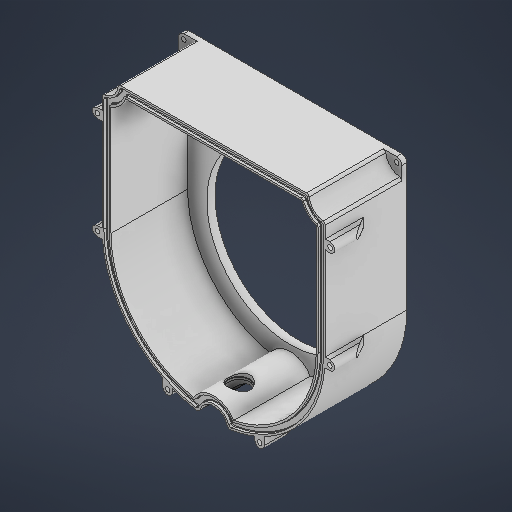
# Autodesk Inventor part: reservoir_cap
Saved by Autodesk Inventor 2026.2 (Build 302298000, 298)
## iProperties
Created: 2026-04-07
Part Number: reservoir_cap
Material: Generic
Document SubType Name: Modeling
Designer: Tathagata Sikdar
Density: 1 g/cm^3
Appearance: Default
Author: Tathagata Sikdar
Autodesk Inventor part; units mm, degrees
note: some values were not read from the file. Chosen so that the rebuilt part matches the saved one: direction of "Hole2".
ref_plane "Work Plane1" through (0, 0, 0) normal (0, 0, 1) x (1, 0, 0)
sketch "Sketch1" plane through (0, 0, 0) normal (0, 0, 1) x (1, 0, 0)
  arc A0 (-87.3944, 0) -> (87.3944, 0) centre (0, 0) ccw projected
  line L0 (-87.3944, 0) -> (-87.3944, 100.0128) projected
  arc A1 (-83.3944, 104.0128) -> (-87.3944, 100.0128) centre (-83.3944, 100.0128) ccw projected
  line L1 (-83.3944, 104.0128) -> (83.3944, 104.0128) projected
  arc A2 (87.3944, 100.0128) -> (83.3944, 104.0128) centre (83.3944, 100.0128) ccw projected
  line L2 (87.3944, 100.0128) -> (87.3944, 0) projected
  circle A3 centre (83.3944, 100.0128) radius 1.85 projected
  circle A4 centre (-83.3944, 100.0128) radius 1.85 projected
  circle A5 centre (0, -83.8944) radius 1.85 projected
  circle A6 centre (0, 0) radius 68.3944 construction
  arc A7 (10, -69.6805) -> (-10, -69.6805) centre (0, 0) ccw construction
  arc A8 (-39.9607, -69.7596) -> (-10, -69.6805) centre (-25.049, -43.7281) ccw construction
  arc A9 (-80.3944, 0) -> (-39.9607, -69.7596) centre (0, 0) ccw construction
  line L3 (-80.3944, 87.0128) -> (-80.3944, 0) construction
  line L4 (-70.3944, 97.0128) -> (-80.3944, 87.0128) construction
  line L5 (70.3944, 97.0128) -> (-70.3944, 97.0128) construction
  line L6 (80.3944, 87.0128) -> (70.3944, 97.0128) construction
  line L7 (80.3944, 0) -> (80.3944, 87.0128) construction
  arc A10 (39.9607, -69.7596) -> (80.3944, 0) centre (0, 0) ccw construction
  arc A11 (10, -69.6805) -> (39.9607, -69.7596) centre (25.049, -43.7281) ccw construction
  arc A12 (14.16, -70.0577) -> (-14.16, -70.0577) centre (0, 0) ccw
  arc A13 (42.1402, -68.1714) -> (80.1444, 0) centre (0, 0) ccw
  line L8 (80.1444, 0) -> (80.1444, 86.9092)
  line L9 (80.1444, 86.9092) -> (70.2909, 96.7628)
  line L10 (70.2909, 96.7628) -> (-70.2909, 96.7628)
  line L11 (-70.2909, 96.7628) -> (-80.1444, 86.9092)
  line L12 (-80.1444, 86.9092) -> (-80.1444, 0)
  arc A14 (-80.1444, 0) -> (-42.1402, -68.1714) centre (0, 0) ccw
  circle A15 centre (0, 0) radius 67.3144
  arc A16 (14.16, -70.0577) -> (42.1402, -68.1714) centre (26.3661, -42.6532) ccw
  arc A17 (-42.1402, -68.1714) -> (-14.16, -70.0577) centre (-26.3661, -42.6532) ccw
  circle A18 centre (0, 0) radius 65.3144
  arc A19 (17.5846, -71.3391) -> (-17.5846, -71.3391) centre (0, 0) ccw
  line L13 (-78.1444, 0) -> (-78.1444, 86.0808)
  line L14 (-78.1444, 86.0808) -> (-69.4624, 94.7628)
  line L15 (-69.4624, 94.7628) -> (69.4624, 94.7628)
  line L16 (69.4624, 94.7628) -> (78.1444, 86.0808)
  line L17 (78.1444, 86.0808) -> (78.1444, 0)
  arc A20 (41.0886, -66.4701) -> (78.1444, 0) centre (0, 0) ccw
  arc A21 (21.565, -70.2385) -> (41.0886, -66.4701) centre (26.3661, -42.6532) ccw
  arc A22 (21.565, -70.2385) -> (-21.565, -70.2385) centre (0, 0) ccw
  arc A23 (-41.0886, -66.4701) -> (-21.565, -70.2385) centre (-26.3661, -42.6532) ccw
  arc A24 (-78.1444, 0) -> (-41.0886, -66.4701) centre (0, 0) ccw
  point P0 (-21.565, -70.2385)
  point P1 (21.565, -70.2385)
  dimension "GasketWidth" = 4.16
  dimension "d1" = 2
  dimension "d2" = -1.08
  dimension "Tolerance" = 0.25
  dimension "d4" = 2
  dimension "d5" = 4.16
  dimension "d6" = 4.16
  dimension "d7" = 2
  dimension "d10" = 2
  constraints: 24 point on circle, 20 end point, 13 centre point, 2 equal radius, 2 tangent, 1 coincident, 15 other
  measures "GasketWidth" radial gap between concentric circles of A12 A15
  measures "d1" radial gap between concentric circles of A7 A6
  measures "d2" radial gap between concentric circles of A6 A15
  measures "Tolerance" distance between parallel lines of L5 L10
  measures "d4" radial gap between concentric circles of A15 A18
  measures "d5" horizontal distance of A7.start A12.start
  measures "d6" horizontal distance of A7.end A12.end
  measures "d7" radial gap between concentric circles of A19 A12
  measures "d10" distance between parallel lines of L12 L13
extrude "Extrusion1" add sketch "Sketch1" against normal blind 2.38 contours A12 A17 A19 A16 | A19 A21 A20 L17 L16 L15 L14 L13 A24 A23 A17 A14 L12 L11 L10 L9 L8 A13 A16 | A15
ref_plane "Work Plane2" through (0, 0, 0) normal (0, 0, 1) x (1, 0, 0)
sketch "Sketch2" plane through (0, 0, 0) normal (0, 0, 1) x (1, 0, 0)
  arc A0 (-87.3944, 0) -> (87.3944, 0) centre (0, 0) ccw projected
  line L0 (-87.3944, 0) -> (-87.3944, 100.0128) projected
  arc A1 (-83.3944, 104.0128) -> (-87.3944, 100.0128) centre (-83.3944, 100.0128) ccw projected
  line L1 (-83.3944, 104.0128) -> (83.3944, 104.0128) projected
  arc A2 (87.3944, 100.0128) -> (83.3944, 104.0128) centre (83.3944, 100.0128) ccw projected
  line L2 (87.3944, 100.0128) -> (87.3944, 0) projected
  circle A3 centre (83.3944, 100.0128) radius 1.85 projected
  circle A4 centre (-83.3944, 100.0128) radius 1.85 projected
  circle A5 centre (0, -83.8944) radius 1.85 projected
  circle A6 centre (0, 0) radius 65.3144 projected
extrude "Extrusion2" add sketch "Sketch2" along normal blind 4
fillet "Fillet1" radius 0.4 2 edges at (-67.3144, 0, 0) (0, 71.4744, 0)
sketch "Sketch3" plane through (0, 0, 4) normal (0, 0, 1) x (1, 0, 0)
  arc A0 (-87.3944, 0) -> (87.3944, 0) centre (0, 0) ccw construction
  line L0 (-87.3944, 100.0128) -> (-87.3944, 0) construction
  arc A1 (-83.3944, 104.0128) -> (-87.3944, 100.0128) centre (-83.3944, 100.0128) ccw construction
  line L1 (83.3944, 104.0128) -> (-83.3944, 104.0128) construction
  arc A2 (87.3944, 100.0128) -> (83.3944, 104.0128) centre (83.3944, 100.0128) ccw construction
  line L2 (87.3944, 0) -> (87.3944, 100.0128) construction
  line L3 (-87.3944, 0) -> (-87.3944, 91.2848)
  line L4 (-74.6665, 104.0128) -> (74.6665, 104.0128)
  line L5 (87.3944, 91.2848) -> (87.3944, 0)
  arc A3 (11.1256, -86.6834) -> (87.3944, 0) centre (0, 0) ccw
  arc A4 (-87.3944, 0) -> (-11.1256, -86.6834) centre (0, 0) ccw
  circle A5 centre (0, -83.8944) radius 1.85 construction
  arc A6 (74.6665, 104.0128) -> (87.3944, 91.2848) centre (87.3944, 104.0128) ccw
  arc A7 (-87.3944, 91.2848) -> (-74.6665, 104.0128) centre (-87.3944, 104.0128) ccw
  arc A8 (11.1256, -86.6834) -> (-11.1256, -86.6834) centre (0, -88.1113) ccw
  line L6 (-74.6665, 104.0128) -> (74.6665, 104.0128)
  arc A9 (74.6665, 104.0128) -> (87.3944, 91.2848) centre (87.3944, 104.0128) ccw
  line L7 (87.3944, 91.2848) -> (87.3944, 0)
  arc A10 (11.1256, -86.6834) -> (87.3944, 0) centre (0, 0) ccw
  arc A11 (11.1256, -86.6834) -> (-11.1256, -86.6834) centre (0, -88.1113) ccw
  arc A12 (-87.3944, 0) -> (-11.1256, -86.6834) centre (0, 0) ccw
  line L8 (-87.3944, 0) -> (-87.3944, 91.2848)
  arc A13 (-87.3944, 91.2848) -> (-74.6665, 104.0128) centre (-87.3944, 104.0128) ccw
  arc A14 (15.6866, -78.8492) -> (-15.6866, -78.8492) centre (0, -88.1113) ccw
  arc A15 (-80.3944, 0) -> (-15.6866, -78.8492) centre (0, 0) ccw
  arc A16 (15.6866, -78.8492) -> (80.3944, 0) centre (0, 0) ccw
  line L9 (80.3944, 0) -> (80.3944, 85.5685)
  arc A17 (68.9502, 97.0128) -> (80.3944, 85.5685) centre (87.3944, 104.0128) ccw
  line L10 (68.9502, 97.0128) -> (-68.9502, 97.0128)
  arc A18 (-80.3944, 85.5685) -> (-68.9502, 97.0128) centre (-87.3944, 104.0128) ccw
  line L11 (-80.3944, 85.5685) -> (-80.3944, 0)
  point P0 (0, -76.8944)
  point P1 (-78.3944, 95.0128)
  point P2 (78.3944, 95.0128)
  dimension "d14" = 7
  dimension "d15" = 5
  dimension "d16" = 5
  dimension "d17" = 7
  dimension "d18" = 7
  dimension "d19" = 7
  dimension "d20" = 7
  dimension "d21" = 7
  dimension "d22" = 7
  constraints: 34 point on circle, 18 end point, 15 centre point, 7 concentric, 4 line through centre, 2 tangent, 2 vertical, 1 collinear, 1 horizontal, 1 vertical alignment, 13 other
  measures "d14" distance of A5.centre point (0, -76.894)
  measures "d15" horizontal distance of A1.centre point (-78.394, 95.013)
  measures "d16" horizontal distance of A2.centre point (78.394, 95.013)
  measures "d17" radial gap between concentric circles of A6 A17
  measures "d18" radial gap between concentric circles of A13 A18
  measures "d19" distance between parallel lines of L6 L10
  measures "d20" distance between parallel lines of L8 L11
  measures "d21" distance between parallel lines of L2 L9
  measures "d22" radial gap between concentric circles of A8 A14
extrude "Extrusion3" add sketch "Sketch3" along normal blind 60
sketch "Sketch4" plane through (0, 0, 64) normal (0, 0, 1) x (1, 0, 0)
  circle A0 centre (-91.1444, -3.7152) radius 1.85
  arc A1 (-91.1444, 0.0348) -> (-91.1444, -7.4652) centre (-91.1444, -3.7152) ccw
  circle A2 centre (91.0687, -3.7152) radius 1.85
  arc A3 (91.0687, -7.4652) -> (91.0687, 0.0348) centre (91.0687, -3.7152) ccw
  circle A4 centre (-36.0427, -83.7152) radius 1.85
  arc A5 (-39.7927, -83.7152) -> (-32.2927, -83.7152) centre (-36.0427, -83.7152) ccw
  circle A6 centre (36.0427, -83.7152) radius 1.85
  arc A7 (32.2927, -83.7152) -> (39.7927, -83.7152) centre (36.0427, -83.7152) ccw
  circle A8 centre (-91.1444, 76.2848) radius 1.85
  arc A9 (-91.1444, 80.0348) -> (-91.1444, 72.5348) centre (-91.1444, 76.2848) ccw
  circle A10 centre (91.1444, 76.2848) radius 1.85
  arc A11 (91.1444, 72.5348) -> (91.1444, 80.0348) centre (91.1444, 76.2848) ccw
  arc A12 (11.1256, -86.6834) -> (87.3944, 0) centre (0, 0) ccw projected
  line L0 (87.3944, 0) -> (87.3944, 91.2848) projected
  arc A13 (74.6665, 104.0128) -> (87.3944, 91.2848) centre (87.3944, 104.0128) ccw construction
  line L1 (74.6665, 104.0128) -> (-74.6665, 104.0128) construction
  arc A14 (-87.3944, 91.2848) -> (-74.6665, 104.0128) centre (-87.3944, 104.0128) ccw construction
  line L2 (-87.3944, 91.2848) -> (-87.3944, 0) projected
  arc A15 (-87.3944, 0) -> (-11.1256, -86.6834) centre (0, 0) ccw projected
  arc A16 (11.1256, -86.6834) -> (-11.1256, -86.6834) centre (0, -88.1113) ccw construction
  arc A17 (15.6866, -78.8492) -> (80.3944, 0) centre (0, 0) ccw construction
  arc A18 (15.6866, -78.8492) -> (-15.6866, -78.8492) centre (0, -88.1113) ccw construction
  arc A19 (-80.3944, 0) -> (-15.6866, -78.8492) centre (0, 0) ccw construction
  line L3 (-80.3944, 0) -> (-80.3944, 85.5685) construction
  arc A20 (-80.3944, 85.5685) -> (-68.9502, 97.0128) centre (-87.3944, 104.0128) ccw construction
  line L4 (-68.9502, 97.0128) -> (68.9502, 97.0128) construction
  arc A21 (68.9502, 97.0128) -> (80.3944, 85.5685) centre (87.3944, 104.0128) ccw construction
  line L5 (80.3944, 85.5685) -> (80.3944, 0) construction
  line L6 (87.3944, 0) -> (87.3944, 91.2848) construction
  line L7 (-87.3944, 91.2848) -> (-87.3944, 0) construction
  line L8 (-91.1444, 80.0348) -> (-87.3944, 80.0348)
  line L9 (-91.1444, 72.5348) -> (-87.3944, 72.5348)
  line L10 (-91.1444, 0.0348) -> (-87.3944, 0.0348)
  line L11 (-91.1444, -7.4652) -> (-87.075, -7.4652)
  line L12 (-39.7927, -83.7152) -> (-39.7927, -77.8095)
  line L13 (-32.2927, -83.7152) -> (-32.2927, -81.2094)
  line L14 (32.2927, -83.7152) -> (32.2927, -81.2094)
  line L15 (39.7927, -83.7152) -> (39.7927, -77.8095)
  line L16 (91.0687, 0.0348) -> (87.3944, 0.0348)
  line L17 (91.0687, -7.4652) -> (87.075, -7.4652)
  line L18 (91.1444, 80.0348) -> (87.3944, 80.0348)
  line L19 (91.1444, 72.5348) -> (87.3944, 72.5348)
  dimension "d25" = 3.7
  dimension "d27" = 3.7
  dimension "d29" = 3.7
  dimension "d31" = 3.7
  dimension "d33" = 3.7
  dimension "d34" = 7.5
  dimension "d35" = 3.7
  dimension "d37" = 15
  dimension "d38" = 80
  dimension "d39" = 80
  constraints: 24 end point, 18 point on circle, 16 tangent, 12 centre point, 10 point on line, 6 coincident, 6 parallel, 5 equal radius, 4 perpendicular, 3 horizontal alignment
  measures "d25" diameter of A0
  measures "d27" diameter of A2
  measures "d29" diameter of A4
  measures "d31" diameter of A6
  measures "d33" diameter of A8
  measures "d34" diameter of A9
  measures "d35" diameter of A10
  measures "d37" vertical distance of L2.start A8.centre
  measures "d38" distance of A8.centre A0.centre
  measures "d39" vertical distance of A0.centre A4.centre
extrude "Extrusion4" add sketch "Sketch4" against normal blind 30
sketch "Sketch5" plane through (0, 0, 34) normal (0, 0, -1) x (-1, 0, 0)
  line L0 (87.3944, 72.5348) -> (91.1444, 72.5348) projected
  arc A0 (91.1444, 72.5348) -> (91.1444, 80.0348) centre (91.1444, 76.2848) ccw projected
  line L1 (91.1444, 80.0348) -> (87.3944, 80.0348) projected
  line L2 (87.3944, 80.0348) -> (87.3944, 72.5348) projected
  circle A1 centre (91.1444, 76.2848) radius 1.85 projected
  line L3 (87.075, -7.4652) -> (91.1444, -7.4652) projected
  arc A2 (91.1444, -7.4652) -> (91.1444, 0.0348) centre (91.1444, -3.7152) ccw projected
  line L4 (91.1444, 0.0348) -> (87.3944, 0.0348) projected
  arc A3 (87.3944, 0) -> (87.3944, 0.0348) centre (-0.0039, 0.0002) ccw projected
  arc A4 (87.075, -7.4652) -> (87.3944, 0) centre (-0.0039, 0.0002) ccw projected
  circle A5 centre (91.1444, -3.7152) radius 1.85 projected
  line L5 (32.2927, -81.2094) -> (32.2927, -83.7152) projected
  arc A6 (32.2927, -83.7152) -> (39.7927, -83.7152) centre (36.0427, -83.7152) ccw projected
  line L6 (39.7927, -83.7152) -> (39.7927, -77.8095) projected
  arc A7 (32.2927, -81.2094) -> (39.7927, -77.8095) centre (0, 0) ccw projected
  circle A8 centre (36.0427, -83.7152) radius 1.85 projected
  line L7 (-39.7927, -77.8095) -> (-39.7927, -83.7152) projected
  arc A9 (-39.7927, -83.7152) -> (-32.2927, -83.7152) centre (-36.0427, -83.7152) ccw projected
  line L8 (-32.2927, -83.7152) -> (-32.2927, -81.2094) projected
  arc A10 (-39.7927, -77.8095) -> (-32.2927, -81.2094) centre (0, 0) ccw projected
  circle A11 centre (-36.0427, -83.7152) radius 1.85 projected
  line L9 (-87.3944, 0.0348) -> (-91.0687, 0.0348) projected
  arc A12 (-91.0687, 0.0348) -> (-91.0687, -7.4652) centre (-91.0687, -3.7152) ccw projected
  line L10 (-91.0687, -7.4652) -> (-87.075, -7.4652) projected
  arc A13 (-87.3944, 0) -> (-87.075, -7.4652) centre (0.0039, 0.0002) ccw projected
  arc A14 (-87.3944, 0.0348) -> (-87.3944, 0) centre (0.0039, 0.0002) ccw projected
  circle A15 centre (-91.0687, -3.7152) radius 1.85 projected
  line L11 (-87.3944, 80.0348) -> (-91.1444, 80.0348) projected
  arc A16 (-91.1444, 80.0348) -> (-91.1444, 72.5348) centre (-91.1444, 76.2848) ccw projected
  line L12 (-91.1444, 72.5348) -> (-87.3944, 72.5348) projected
  line L13 (-87.3944, 72.5348) -> (-87.3944, 80.0348) projected
  circle A17 centre (-91.1444, 76.2848) radius 1.85 projected
extrude "Extrusion5" add sketch "Sketch5" against normal blind 15 contours L2 L1 A0 L0 | A1 | A4 A3 L4 A2 L3 | A5 | A7 L6 A6 L5 | A8 | A10 L8 A9 L7 | A11 | A14 A13 L10 A12 L9 | A15 | L13 L12 A16 L11 | A17
sketch "Sketch6" plane through (-91.1444, 80.0348, 64) normal (0, 1, 0) x (1, 0, 0)
  line L0 (0, 30) -> (3.75, 30) projected
  line L1 (3.75, 30) -> (-3.75, 17.0096)
  line L2 (-3.75, 0) -> (-3.75, 30) projected
  line L3 (0, 30) -> (-3.75, 30) projected
  line L4 (-3.75, 30) -> (0, 30)
  line L5 (186.0389, 30) -> (182.2889, 30) projected
  line L6 (178.5389, 30) -> (182.2889, 30) projected
  line L7 (186.0389, 0) -> (186.0389, 30) projected
  line L8 (178.5389, 30) -> (186.0389, 17.0096)
  line L9 (-3.75, 17.0096) -> (-4.75, 17.0096)
  line L10 (-4.75, 17.0096) -> (-4.75, 30)
  line L11 (-4.75, 30) -> (-3.75, 30)
  point P0 (91.1444, 64)
  dimension "d44" = 60
  dimension "d45" = 60
  dimension "d48" = 1
  constraints: 12 end point, 2 collinear, 2 horizontal alignment, 2 point on line, 1 horizontal, 1 perpendicular
  measures "d44" angle of L3 L1
  measures "d45" angle of L6 L8
  measures "d48" distance between parallel lines of L2 L10
sketch3d "3D Sketch1"
  line L0 (-87.3944, 100.0128, 0) -> (-87.3944, 0, 0)
  arc A0 (-87.3944, 0, 0) -> (-61.7972, -61.7972, 0) centre (0, 0, 0) ccw
  arc A1 (-61.7972, -61.7972, 0) -> (0, -87.3944, 0) centre (0, 0, 0) ccw
  arc A2 (0, -87.3944, 0) -> (61.7972, -61.7972, 0) centre (0, 0, 0) ccw
  arc A3 (61.7972, -61.7972, 0) -> (87.3944, 0, 0) centre (0, 0, 0) ccw
  line L1 (87.3944, 0, 0) -> (87.3944, 100.0128, 0)
  arc A4 (87.3944, 100.0128, 0) -> (83.3944, 104.0128, 0) centre (83.3944, 100.0128, 0) ccw
  line L2 (83.3944, 104.0128, 0) -> (-83.3944, 104.0128, 0)
  arc A5 (-83.3944, 104.0128, 0) -> (-87.3944, 100.0128, 0) centre (-83.3944, 100.0128, 0) ccw
sweep "Sweep1" cut profiles "Sketch6" path "3D Sketch1" contours L0 L1 L2 L3 | L2 L9 L10 L11
sketch "Sketch7" plane through (0, 0, 64) normal (0, 0, 1) x (1, 0, 0)
  circle A0 centre (91.0687, -3.7152) radius 1.85 construction
  circle A1 centre (-91.1444, -3.7152) radius 1.85 construction
  circle A2 centre (-91.1444, 76.2848) radius 1.85 construction
  circle A3 centre (36.0427, -83.7152) radius 1.85 construction
  circle A4 centre (91.1444, 76.2848) radius 1.85 construction
  circle A5 centre (-36.0427, -83.7152) radius 1.85 construction
  arc A6 (11.1256, -86.6834) -> (32.2927, -81.2094) centre (0, 0) ccw construction
  line L0 (32.2927, -81.2094) -> (32.2927, -83.7152) construction
  arc A7 (32.2927, -83.7152) -> (39.7927, -83.7152) centre (36.0427, -83.7152) ccw construction
  line L1 (39.7927, -83.7152) -> (39.7927, -77.8095) construction
  arc A8 (39.7927, -77.8095) -> (87.075, -7.4652) centre (0, 0) ccw construction
  line L2 (87.075, -7.4652) -> (91.0687, -7.4652) construction
  arc A9 (91.0687, -7.4652) -> (91.0687, 0.0348) centre (91.0687, -3.7152) ccw construction
  line L3 (91.0687, 0.0348) -> (87.3944, 0.0348) construction
  line L4 (87.3944, 0.0348) -> (87.3944, 72.5348) construction
  line L5 (87.3944, 72.5348) -> (91.1444, 72.5348) construction
  arc A10 (91.1444, 72.5348) -> (91.1444, 80.0348) centre (91.1444, 76.2848) ccw construction
  line L6 (91.1444, 80.0348) -> (87.3944, 80.0348) construction
  line L7 (87.3944, 80.0348) -> (87.3944, 91.2848) construction
  arc A11 (74.6665, 104.0128) -> (87.3944, 91.2848) centre (87.3944, 104.0128) ccw construction
  line L8 (74.6665, 104.0128) -> (-74.6665, 104.0128) construction
  arc A12 (-87.3944, 91.2848) -> (-74.6665, 104.0128) centre (-87.3944, 104.0128) ccw construction
  line L9 (-87.3944, 91.2848) -> (-87.3944, 80.0348) construction
  line L10 (-87.3944, 80.0348) -> (-91.1444, 80.0348) construction
  arc A13 (-91.1444, 80.0348) -> (-91.1444, 72.5348) centre (-91.1444, 76.2848) ccw construction
  line L11 (-91.1444, 72.5348) -> (-87.3944, 72.5348) construction
  line L12 (-87.3944, 72.5348) -> (-87.3944, 0.0348) construction
  line L13 (-87.3944, 0.0348) -> (-91.1444, 0.0348) construction
  arc A14 (-91.1444, 0.0348) -> (-91.1444, -7.4652) centre (-91.1444, -3.7152) ccw construction
  line L14 (-91.1444, -7.4652) -> (-87.075, -7.4652) construction
  arc A15 (-87.075, -7.4652) -> (-39.7927, -77.8095) centre (0, 0) ccw construction
  line L15 (-39.7927, -77.8095) -> (-39.7927, -83.7152) construction
  arc A16 (-39.7927, -83.7152) -> (-32.2927, -83.7152) centre (-36.0427, -83.7152) ccw construction
  line L16 (-32.2927, -83.7152) -> (-32.2927, -81.2094) construction
  arc A17 (-32.2927, -81.2094) -> (-11.1256, -86.6834) centre (0, 0) ccw construction
  arc A18 (11.1256, -86.6834) -> (-11.1256, -86.6834) centre (0, -88.1113) ccw construction
  arc A19 (15.6866, -78.8492) -> (80.3944, 0) centre (0, 0) ccw construction
  arc A20 (15.6866, -78.8492) -> (-15.6866, -78.8492) centre (0, -88.1113) ccw construction
  arc A21 (-80.3944, 0) -> (-15.6866, -78.8492) centre (0, 0) ccw construction
  line L17 (-80.3944, 0) -> (-80.3944, 85.5685) construction
  arc A22 (-80.3944, 85.5685) -> (-68.9502, 97.0128) centre (-87.3944, 104.0128) ccw construction
  line L18 (-68.9502, 97.0128) -> (68.9502, 97.0128) construction
  arc A23 (68.9502, 97.0128) -> (80.3944, 85.5685) centre (87.3944, 104.0128) ccw construction
  line L19 (80.3944, 85.5685) -> (80.3944, 0) construction
  arc A24 (14.2722, -79.2546) -> (-14.2722, -79.2546) centre (0, -88.1113) ccw
  arc A25 (16.3718, -80.1596) -> (81.8144, 0) centre (0, 0) ccw
  line L20 (81.8144, 0) -> (81.8144, 85.1725)
  arc A26 (70.4096, 97.1793) -> (80.5609, 87.028) centre (87.3944, 104.0128) ccw
  line L21 (68.5542, 98.4328) -> (-68.5542, 98.4328)
  arc A27 (-80.5609, 87.028) -> (-70.4096, 97.1793) centre (-87.3944, 104.0128) ccw
  line L22 (-81.8144, 85.1725) -> (-81.8144, 0)
  arc A28 (-81.8144, 0) -> (-16.3718, -80.1596) centre (0, 0) ccw
  arc A29 (11.7942, -83.5739) -> (-11.7942, -83.5739) centre (0, -88.1113) ccw
  arc A30 (13.9862, -84.8292) -> (85.9744, 0) centre (0, 0) ccw
  line L23 (85.9744, 0) -> (85.9744, 88.2312)
  arc A31 (73.5675, 101.0163) -> (84.398, 90.1858) centre (87.3944, 104.0128) ccw
  line L24 (71.6128, 102.5928) -> (-71.6128, 102.5928)
  arc A32 (-84.398, 90.1858) -> (-73.5675, 101.0163) centre (-87.3944, 104.0128) ccw
  line L25 (-85.9744, 88.2312) -> (-85.9744, 0)
  arc A33 (-85.9744, 0) -> (-13.9862, -84.8292) centre (0, 0) ccw
  arc A34 (70.4096, 97.1793) -> (68.5542, 98.4328) centre (68.5542, 96.4328) ccw
  arc A35 (73.5675, 101.0163) -> (71.6128, 102.5928) centre (71.6128, 100.5928) ccw
  arc A36 (85.9744, 88.2312) -> (84.398, 90.1858) centre (83.9744, 88.2312) ccw
  arc A37 (81.8144, 85.1725) -> (80.5609, 87.028) centre (79.8144, 85.1725) ccw
  arc A38 (-68.5542, 98.4328) -> (-70.4096, 97.1793) centre (-68.5542, 96.4328) ccw
  arc A39 (-71.6128, 102.5928) -> (-73.5675, 101.0163) centre (-71.6128, 100.5928) ccw
  arc A40 (-84.398, 90.1858) -> (-85.9744, 88.2312) centre (-83.9744, 88.2312) ccw
  arc A41 (-80.5609, 87.028) -> (-81.8144, 85.1725) centre (-79.8144, 85.1725) ccw
  arc A42 (-16.3718, -80.1596) -> (-14.2722, -79.2546) centre (-15.9716, -78.2001) ccw
  arc A43 (-13.9862, -84.8292) -> (-11.7942, -83.5739) centre (-13.6608, -82.8558) ccw
  arc A44 (14.2722, -79.2546) -> (16.3718, -80.1596) centre (15.9716, -78.2001) ccw
  arc A45 (11.7942, -83.5739) -> (13.9862, -84.8292) centre (13.6608, -82.8558) ccw
  point P0 (81.8144, 86.5759)
  point P1 (69.9576, 98.4328)
  point P2 (-69.9576, 98.4328)
  point P3 (-81.8144, 86.5759)
  point P4 (85.9744, 89.9363)
  point P5 (73.3179, 102.5928)
  point P6 (-73.3179, 102.5928)
  point P7 (-85.9744, 89.9363)
  dimension "d49" = 4.16
  dimension "d50" = 7
  dimension "d51" = 1.42
  dimension "d52" = 2
  constraints: 52 point on circle, 24 tangent, 22 centre point, 12 end point, 11 equal radius, 8 point on line, 14 other
  measures "d49" radial gap between concentric circles of A33 A28
  measures "d50" radial gap between concentric circles of A15 A21
  measures "d51" radial gap between concentric circles of A28 A21
  measures "d52" radius of A34
extrude "Extrusion6" cut sketch "Sketch7" against normal blind 2.38
fillet "Fillet2" radius 0.4 28 edges at (-85.5312, 89.4867, 61.62) (-77.3903, 94.0087, 61.62) (-72.8684, 102.1495, 61.62) (0, 102.5928, 61.62) (72.8684, 102.1495, 61.62) (77.3903, 94.0087, 61.62) (85.5312, 89.4867, 61.62) (85.9744, 44.1156, 61.62) (65.5517, -55.6289, 61.62) (12.667, -84.5914, 61.62) (0, -75.4744, 61.62) (-12.667, -84.5914, 61.62) (-65.5517, -55.6289, 61.62) (-85.9744, 44.1156, 61.62) (-63.3761, -51.7405, 61.62) (-15.1799, -80.0367, 61.62) (0, -71.3144, 61.62) (15.1799, -80.0367, 61.62) (63.3761, -51.7405, 61.62) (81.8144, 42.5863, 61.62) (81.4717, 86.2921, 61.62) (74.4488, 91.0671, 61.62) (69.6738, 98.09, 61.62) (0, 98.4328, 61.62) (-69.6738, 98.09, 61.62) (-74.4488, 91.0671, 61.62) (-81.4717, 86.2921, 61.62) (-81.8144, 42.5863, 61.62)
fillet "Fillet3" radius 2 6 edges at (-87.3944, 91.2848, 34) (-74.6665, 104.0128, 34) (74.6665, 104.0128, 34) (87.3944, 91.2848, 34) (11.1256, -86.6834, 34) (-11.1256, -86.6834, 34)
sketch "Sketch8" plane through (0, 0, 4) normal (0, 0, 1) x (1, 0, 0)
  circle A0 centre (0, 0) radius 65.3144 projected
  line L0 (0, 65.3144) -> (50, 65.3144) construction
  line L1 (50, 65.3144) -> (64.1421, 51.1723) construction
  point P0 (64.1421, 51.1723)
  dimension "d58" = 50
  dimension "d67" = 20
  dimension "d69" = 135
  constraints: 4 end point, 2 horizontal, 1 coincident, 1 vertical alignment, 1 other
  measures "d58" distance of L0.start L0.end
  measures "d67" distance of L0.end L1.end
  measures "d69" angle of L0 L1
hole "Hole1" at (64.1421, 51.1723, 4) direction (0, 0, -1) diameter 16 end through all
ref_plane "Work Plane3" through (-12.9956, -86.4228, 0) normal (0, -1, 0) x (0, 0, -1)
sketch "Sketch9" plane through (-12.9956, -86.4228, 0) normal (0, -1, 0) x (0, 0, -1)
  line L0 (-64, 23.7723) -> (-4, 23.7723) construction
  line L1 (-4, 2.2189) -> (-64, 2.2189) construction
  line L2 (-64, 2.2189) -> (-64, 23.7723) construction
  line L3 (-64, 12.9956) -> (-44, 12.9956) construction
  point P0 (0, 12.9956)
  dimension "d71" = 20
  constraints: 4 end point, 2 perpendicular, 1 coincident, 1 midpoint, 1 point on line
  measures "d71" distance of L3.start L3.end
hole "Hole2" at (0, -86.4228, 44) direction (0, 1, 0) diameter 16 end up to surface
hole "Hole3" at (0, -86.4228, 44) direction (0, 1, 0) diameter 17 depth 12
ref_plane "Work Plane4" through (0, -69.8944, 4) normal (0, -1, 0) x (0, 0, -1)
sketch "Sketch11" plane through (0, -69.8944, 4) normal (0, -1, 0) x (0, 0, -1)
  point P0 (4, 0)
  point P1 (-40, 0)
hole "Hole4" at (0, -69.8944, 44) direction (0, -1, 0) diameter 17 depth 3
equation "\"d2\" = -0.5 * GasketWidth + 0.5 * d1"
equation "\"d5\" = GasketWidth"
equation "\"d6\" = GasketWidth"
equation "\"d18\" = d17"
equation "\"d19\" = d17"
equation "\"d20\" = d17"
equation "\"d21\" = d17"
equation "\"d22\" = d17"
equation "\"d51\" = -0.5 * d49 + 0.5 * d50"
body "Solid1"
